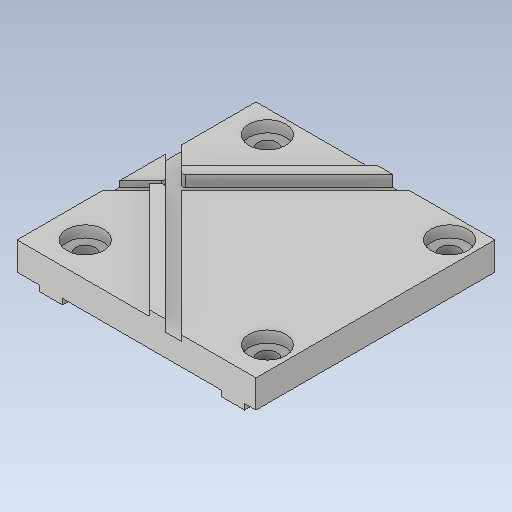
# Autodesk Inventor part: FAB-OX0006
Saved by Autodesk Inventor 2020 (Build 240168000, 168)
## iProperties
Created: 2017-01-09
Part Number: FAB-OX0006
Material: Generic
Document SubType Name: Modeling
Designer: map
Density: 1 g/cm^3
Appearance: Default
Description: Goniometer cube mount
Author: map
Revision Number: 02
Autodesk Inventor part; units mm, degrees
ref_plane "YZ Plane" through (0, 0, 0) normal (1, 0, 0) x (0, 1, 0)
ref_plane "XZ Plane" through (0, 0, 0) normal (0, 1, 0) x (-1, 0, 0)
ref_plane "XY Plane" through (0, 0, 0) normal (0, 0, 1) x (1, 0, 0)
sketch "Sketch1" plane through (0, 0, 0) normal (0, 1, 0) x (-1, 0, 0)
  line L0 (20, 20) -> (-20, 20)
  line L1 (-20, 20) -> (-20, -20)
  line L2 (-20, -20) -> (20, -20)
  line L3 (20, -20) -> (20, 20)
  line L4 (20, 20) -> (-20, -20) construction
  point P0 (0, 0)
  point P1 (0, 0)
  dimension "d6" = 40
  dimension "d7" = 40
  constraints: 10 end point, 2 parallel, 1 coincident, 1 horizontal, 1 midpoint, 1 perpendicular
  measures "d6" distance of L2.end L1.end
  measures "d7" distance of L1.end L0.end
extrude "Extrusion2" add sketch "Sketch1" along normal blind 4.9
sketch "Sketch2" plane through (0, 4.9, 0) normal (0, 1, 0) x (1, 0, 0)
  line L0 (-19.8943, 8.5431) -> (-13.3498, 8.5431) construction
  line L1 (-16.5463, 1.4142) -> (2.0395, 20)
  line L2 (20, 20) -> (-20, 20) projected
  line L3 (-20, 20) -> (-20, -20) projected
  line L4 (-20, 0) -> (20, 0)
  line L5 (20, -20) -> (20, 20) projected
  line L6 (-16.5463, 1.4142) -> (-17.9605, 2.8284)
  line L7 (-17.9605, 2.8284) -> (-0.7889, 20)
  line L8 (-16.5463, -1.4142) -> (2.0395, -20)
  line L9 (20, -20) -> (-20, -20)
  line L10 (-16.5463, -1.4142) -> (-17.9605, -2.8284)
  line L11 (-17.9605, -2.8284) -> (-0.7889, -20)
  line L12 (-16.5463, 1.4142) -> (-12.694, -2.4381) construction
  point P0 (0, 0)
  dimension "d17" = 12.7
  dimension "d18" = 135
  dimension "d19" = 2
  dimension "d51" = 2
  constraints: 20 end point, 4 point on line, 4 symmetric about line, 2 midpoint, 1 horizontal, 1 parallel, 1 perpendicular
  measures "d17" distance from line of L1 point (0, 0)
  measures "d18" angle of L2 L1
  measures "d19" distance of L1.start L6.end
  measures "d51" distance between parallel lines of L12 L8
extrude "Extrusion3" add sketch "Sketch2" along normal blind 1 contours L6 L7 L2 L1 | L9 L11 L10 L8
sketch "Sketch3" plane through (0, 4.9, 0) normal (0, 1, 0) x (1, 0, 0)
  line L0 (-20, -20) -> (-20, 20) construction
  line L1 (-20, 20) -> (-0.7889, 20) construction
  line L2 (-17.9605, 2.8284) -> (-0.7889, 20) construction
  line L3 (-16.5463, 1.4142) -> (-17.9605, 2.8284) construction
  line L4 (2.0395, 20) -> (-16.5463, 1.4142) construction
  line L5 (2.0395, 20) -> (20, 20) construction
  line L6 (20, 20) -> (20, -20) construction
  line L7 (20, -20) -> (2.0395, -20) construction
  line L8 (2.0395, -20) -> (-0.7889, -20) construction
  line L9 (-0.7889, -20) -> (-20, -20) construction
  line L10 (-0.7889, 20) -> (2.0395, 20) construction
  line L11 (-16.5463, -1.4142) -> (2.0395, -20) construction
  line L12 (-17.9605, -2.8284) -> (-16.5463, -1.4142) construction
  line L13 (-0.7889, -20) -> (-17.9605, -2.8284) construction
  line L14 (2.0395, -20) -> (20, -20) projected
  line L15 (-20, 20) -> (-20, -20) projected
  line L16 (20, 20) -> (2.0395, 20) projected
  line L17 (-17.9605, 2.8284) -> (-16.5463, 1.4142) projected
  line L18 (2.0395, 20) -> (-16.5463, 1.4142)
  line L19 (-17.9605, 0) -> (-20, -2.0395)
  line L20 (2.0395, -20) -> (-16.5463, -1.4142)
  line L21 (-17.9605, 0) -> (-20, 2.0395)
  line L22 (2.0395, -20) -> (-16.5463, -1.4142) projected
  line L23 (-16.5463, 1.4142) -> (2.0395, 20) projected
  line L24 (4.8679, -20) -> (-15.1321, 0)
  line L25 (-16.5463, 1.4142) -> (-20, 4.8679)
  line L26 (-20, -4.8679) -> (-16.5463, -1.4142)
  line L27 (-15.1321, 0) -> (4.8679, 20)
  line L28 (-20, -2.0395) -> (-20, -4.8679)
  line L29 (-20, 2.0395) -> (-20, 4.8679)
  constraints: 22 end point, 10 perpendicular, 7 collinear, 7 point on line, 1 vertical
extrude "Extrusion4" cut sketch "Sketch3" against normal blind 1 contours L20 L26 L15 L19 L21 L25 L17 L18 L16 L27 L24 L14
sketch "Sketch4" plane through (0, 4.9, 0) normal (0, 1, 0) x (1, 0, 0)
  line L0 (16, -16) -> (-16, -16)
  line L1 (-16, -16) -> (-16, 16)
  line L2 (-16, 16) -> (16, 16)
  line L3 (16, 16) -> (16, -16)
  line L4 (16, -16) -> (-16, 16) construction
  line L5 (-16, -16) -> (16, 16) construction
  point P0 (0, 0)
  dimension "d27" = 32
  dimension "d28" = 32
  constraints: 12 end point, 7 coincident, 2 midpoint, 2 parallel, 1 horizontal, 1 perpendicular
  measures "d27" distance of L1.end L2.end
  measures "d28" distance of L0.end L1.end
hole "Hole1" at (-16, 4.9, -16) at (16, 4.9, -16) at (16, 4.9, 16) at (-16, 4.9, 16) direction (0, -1, 0) diameter 3.4 end through all counterbore diameter 6.5 counterbore depth 2 clearance for "Socket Head Cap Screw ISO 4762" size "M3" standard "ISO"
move faces "Move1" translate (-2, 0, 0) faces at (-20, 1.3, -1.6226)
move faces "Move2" translate (0, 0, 2) faces at (0.0132, 1.3, 20)
sketch "Sketch5" plane through (0, 0, 0) normal (0, -1, 0) x (1, 0, 0)
  line L0 (-22, -20) -> (-22, 22) construction
  line L1 (-0.7889, -20) -> (-22, -20) projected
  line L2 (-22, 22) -> (-20, 22) construction
  line L3 (-20, 20) -> (-20, -20) construction
  line L4 (-20, -20) -> (-22, -20) construction
  line L5 (-22, -20) -> (-22, 22) construction
  line L6 (-22, 22) -> (20, 22) construction
  line L7 (20, 22) -> (20, -20) construction
  line L8 (-22, 22) -> (20, 22) construction
  line L9 (20, 22) -> (20, 20) construction
  line L10 (20, 20) -> (-20, 20) construction
  line L11 (-22, 20) -> (-22, 22) construction
  line L12 (-22, 22) -> (1.2111, 22) construction
  line L13 (-14, 22) -> (-18, 22)
  line L14 (-18, 22) -> (-18, 20)
  line L15 (-18, 20) -> (-14, 20)
  line L16 (-14, 20) -> (-14, 22)
  line L17 (18, 20) -> (14, 20)
  line L18 (14, 20) -> (14, 22)
  line L19 (14, 22) -> (18, 22)
  line L20 (18, 22) -> (18, 20)
  line L21 (0, 0) -> (0, 24.7178)
  line L22 (-20, 14) -> (-22, 14)
  line L23 (-22, 14) -> (-22, 18)
  line L24 (-22, 18) -> (-20, 18)
  line L25 (-20, 18) -> (-20, 14)
  line L26 (-20, -18) -> (-22, -18)
  line L27 (-22, -18) -> (-22, -14)
  line L28 (-22, -14) -> (-20, -14)
  line L29 (-20, -14) -> (-20, -18)
  line L30 (0, 0) -> (-29.8297, 0)
  dimension "d42" = 2
  dimension "d43" = 2
  dimension "d46" = 28
  dimension "d47" = 4
  dimension "d49" = 4
  dimension "d50" = 28
  constraints: 52 end point, 12 parallel, 9 point on line, 7 horizontal, 6 perpendicular, 1 collinear, 1 vertical, 4 other
  measures "d42" distance of L3.end L4.end
  measures "d43" distance of L8.end L9.end
  measures "d46" diameter of L18 L21
  measures "d47" distance of L18.end L19.end
  measures "d49" distance of L22.end L23.end
  measures "d50" distance between parallel lines of L28 L22
extrude "Extrusion5" add sketch "Sketch5" along normal blind 1
fillet "Fillet2" radius 0.5 3 edges at (-16.5463, 4.9, -1.4142) (-17.9605, 4.4, 0) (-16.5463, 4.9, 1.4142)
equation "\"d6\" = edge"
equation "\"d7\" = edge"
equation "\"d14\" = workingThickness"
equation "\"d17\" = 0.5 * cubeEdge"
equation "\"d19\" = 2 * upstand"
equation "\"d21\" = upstand"
equation "\"d25\" = glueGrooveDepth"
equation "\"d27\" = holePatternEdge"
equation "\"d28\" = d27"
equation "\"d44\" = upstand"
equation "\"edge\" = 40"
equation "\"holePatternEdge\" = 32"
equation "\"workingThickness\" = 4.9"
equation "\"cubeEdge\" = 25.4"
equation "\"upstand\" = 1"
equation "\"glueGrooveDepth\" = 1"
body "Solid2"
